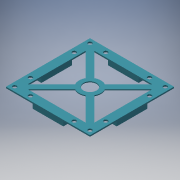
# Autodesk Inventor part: Base
Saved by Autodesk Inventor 2016 (Build 200138000, 138)
## iProperties
Created: 2015-03-29
Part Number: Base
Material: PC/ABS Plastic
Document SubType Name: Modeling
Designer: Erin
Density: 0.357273 g/cm^3
Appearance: Cadet Blue
Mass: 3.14413 g
Surface Area: 66.4965 cm^2
Volume: 5.71659 cm^3
Author: Erin
Autodesk Inventor part; units mm, degrees
ref_plane "YZ Plane" through (0, 0, 0) normal (1, 0, 0) x (0, 1, 0)
ref_plane "XZ Plane" through (0, 0, 0) normal (0, 1, 0) x (-1, 0, 0)
ref_plane "XY Plane" through (0, 0, 0) normal (0, 0, 1) x (1, 0, 0)
sketch "Sketch1" plane through (0, 0, 0) normal (0, 0, 1) x (1, 0, 0)
  line L0 (-48, 48) -> (48, 48)
  line L1 (48, 48) -> (48, -48)
  line L2 (48, -48) -> (-48, -48)
  line L3 (-48, -48) -> (-48, 48)
  line L4 (38, 38) -> (-38, 38)
  line L5 (-38, 38) -> (-38, -38)
  line L6 (-38, -38) -> (38, -38)
  line L7 (38, -38) -> (38, 38)
  line L8 (0, 152.7233) -> (0, -72.1628) construction
  line L9 (-77.8847, 0) -> (88.8171, 0) construction
  line L10 (-48, 43) -> (48, 43) construction
  line L11 (-43, 48) -> (-43, -48) construction
  line L12 (-48, -43) -> (48, -43) construction
  circle A0 centre (-43, 25) radius 2.25
  circle A1 centre (-43, -25) radius 2.25
  circle A2 centre (-43, -43) radius 2.25
  circle A3 centre (-43, 43) radius 2.25
  line L13 (-48, 30) -> (48, 30) construction
  line L14 (-48, -30) -> (48, -30) construction
  line L15 (-50, 31) -> (-36, 31)
  line L16 (-36, 31) -> (-36, -31)
  line L17 (-36, -31) -> (-50, -31)
  line L18 (-50, -31) -> (-50, 31)
  point P0 (0, 0)
  point P1 (0, 48)
  point P2 (48, 0)
  dimension "d0" = 96
  dimension "d1" = 96
  dimension "d2" = 10
  dimension "d5" = 5
  dimension "d11" = 5
  dimension "d14" = 5
  dimension "d31" = 4.5
  dimension "d32" = 4.5
  dimension "d61" = 4.5
  dimension "d62" = 4.5
  dimension "d65" = 30
  dimension "d66" = 30
  dimension "d67" = 5
  dimension "d68" = 5
  dimension "d74" = 1
  dimension "d75" = 1
  dimension "d76" = 2
  dimension "d77" = 2
  constraints: 38 end point, 16 point on line, 9 perpendicular, 7 parallel, 4 centre point, 3 horizontal, 2 midpoint, 1 horizontal alignment, 1 vertical, 1 vertical alignment, 3 other
  measures "d0" distance of L1.end L2.end
  measures "d1" distance of L0.end L1.end
  measures "d2" distance between parallel lines of L4 L0
  measures "d5" distance between parallel lines of L10 L0
  measures "d11" distance between parallel lines of L11 L3
  measures "d14" distance between parallel lines of L12 L2
  measures "d31" diameter of A0
  measures "d32" diameter of A1
  measures "d61" diameter of A2
  measures "d62" diameter of A3
  measures "d65" distance between parallel lines of L13 L9
  measures "d66" distance between parallel lines of L14 L9
  measures "d67" distance from line of A1.centre L14
  measures "d68" distance from line of A0.centre L13
  measures "d74" distance between parallel lines of L13 L15
  measures "d75" distance between parallel lines of L17 L14
  measures "d76" distance between parallel lines of L3 L18
  measures "d77" distance between parallel lines of L16 L5
extrude "Extrusion1" add sketch "Sketch1" against normal blind 1.5 contours L0 L1 L2 L3 L17 L5 L6 L7 L4 L15 | L15 L5 L17 L3 | A0 | A1 | A2 | A3
extrude "Extrusion2" cut sketch "Sketch1" against normal blind 10 contours A2 | A3
mirror "Mirror5" about plane through (0, 0, 0) normal (1, 0, 0) of "Extrusion2"
extrude "Extrusion5" cut sketch "Sketch1" against normal blind 10 contours A0 | A1
pattern_circular "Circular Pattern1" count 4 over 360 about axis through (0, 0, -10) along (0, 0, 1) of "Extrusion5"
sketch "Sketch3" plane through (0, 0, 0) normal (0, 0, 1) x (1, 0, 0)
  circle A0 centre (25, 43) radius 2.25 projected
  circle A1 centre (-25, 43) radius 2.25 projected
  circle A2 centre (43, -25) radius 2.25 projected
  circle A3 centre (43, 25) radius 2.25 projected
  circle A4 centre (-25, -43) radius 2.25 projected
  circle A5 centre (25, -43) radius 2.25 projected
  circle A6 centre (-43, 25) radius 2.25 projected
  circle A7 centre (-43, -25) radius 2.25 projected
  circle A8 centre (43, -43) radius 2.25 projected
  circle A9 centre (43, 43) radius 2.25 projected
  circle A10 centre (-43, -43) radius 2.25 projected
  circle A11 centre (-43, 43) radius 2.25 projected
  line L0 (-38, -38) -> (-38, 38) projected
  line L1 (-38, 38) -> (38, 38) projected
  line L2 (38, 38) -> (38, -38) projected
  line L3 (38, -38) -> (-38, -38) projected
  line L4 (-48, 48) -> (48, 48) projected
  line L5 (-48, -48) -> (-48, 48) projected
  line L6 (48, -48) -> (-48, -48) projected
  line L7 (48, 48) -> (48, -48) projected
  circle A12 centre (0, 0) radius 7.5
  circle A13 centre (0, 0) radius 12.5
  line L8 (-35.5251, 40.4749) -> (40.4749, -35.5251)
  line L9 (40.4749, -35.5251) -> (35.5251, -40.4749)
  line L10 (35.5251, -40.4749) -> (-40.4749, 35.5251)
  line L11 (-40.4749, 35.5251) -> (-35.5251, 40.4749)
  line L12 (-38, 38) -> (38, -38) construction
  line L13 (2.4749, 2.4749) -> (-2.4749, -2.4749) construction
  dimension "d80" = 15
  dimension "d81" = 5
  dimension "d82" = 7
  constraints: 12 end point, 5 midpoint, 3 coincident, 2 centre point, 2 parallel, 1 perpendicular
  measures "d80" diameter of A12
  measures "d81" radial gap between concentric circles of A12 A13
  measures "d82" distance of L8.end L9.end
extrude "Extrusion7" add sketch "Sketch3" against normal blind 1 contours L10 A12 A13 | A13 L8 A12 L10 | L10 A12 L8 A13 | A13 L8 A12
extrude "Extrusion8" add sketch "Sketch3" against normal blind 1 contours L10 L11 L0 | L0 L1 L8 A13 L10 | L10 A13 L8 L2 L3 | L3 L9 L10 | L11 L8 L1 | A13 L8 A12 L10 | L2 L8 L9 | L10 A12 L8 A13 | A12 L8 L10
mirror "Mirror6" about plane through (0, 0, 0) normal (1, 0, 0) of "Extrusion8"
extrude "Extrusion9" cut sketch "Sketch3" against normal blind 1 contours L10 A12 | A12 L8 L10 | A12 L8
sketch "Sketch4" plane through (0, 0, -1.5) normal (0, 0, -1) x (-1, 0, 0)
  line L0 (48, -48) -> (48, 48) projected
  line L1 (38, -33.0503) -> (38, 33.0503) projected
  line L2 (48, -17.5) -> (38, -17.5)
  line L3 (38, -17.5) -> (38, 17.5)
  line L4 (38, 17.5) -> (48, 17.5)
  line L5 (48, 17.5) -> (48, -17.5)
  point P0 (0, 0)
  point P1 (38, 0)
  point P2 (38, 0)
  dimension "d89" = 35
  constraints: 8 end point, 2 midpoint, 2 parallel, 2 point on line, 1 coincident, 1 horizontal, 1 perpendicular
  measures "d89" distance between parallel lines of L4 L2
extrude "Extrusion10" add sketch "Sketch4" along normal blind 5
pattern_circular "Circular Pattern2" count 4 over 360 about axis through (0, 0, -10) along (0, 0, 1) of "Extrusion10"
equation "\"d31\" = screw"
equation "\"d32\" = screw"
equation "\"d61\" = screw"
equation "\"d62\" = screw"
equation "\"screw\" = 4.5"
body "Solid1"
